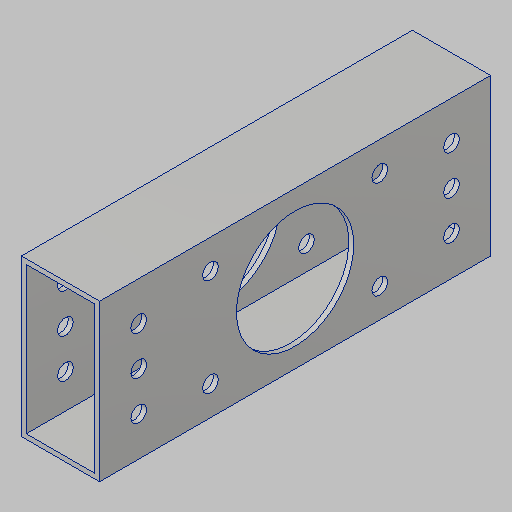
# Autodesk Inventor part: GP5-001
Saved by Autodesk Inventor 2023.4 (Build 274418000, 418)
## iProperties
RuleStatus: InUse
Created: 2025-01-28
Part Number: GP5-001
Material: Aluminum 6061
Document SubType Name: Modeling
Designer: slick
Mass: 304.185 g
Surface Area: 718.547 cm^2
Volume: 112.661 cm^3
Density: 2.7 g/cm^3
Appearance: Aluminum - Flat
AfterDocNew0: SHOW
AfterDocOpen0: SHOW
Author: slick
Autodesk Inventor part; units mm, degrees
ref_plane "YZ Plane" through (0, 0, 0) normal (1, 0, 0) x (0, 1, 0)
ref_plane "XZ Plane" through (0, 0, 0) normal (0, 1, 0) x (-1, 0, 0)
ref_plane "XY Plane" through (0, 0, 0) normal (0, 0, 1) x (1, 0, 0)
sketch "Sketch1" plane through (0, 0, 0) normal (0, 0, 1) x (1, 0, 0)
  line L0 (-12.7, -25.4) -> (12.7, -25.4)
  line L1 (12.7, -25.4) -> (12.7, 25.4)
  line L2 (12.7, 25.4) -> (-12.7, 25.4)
  line L3 (-12.7, 25.4) -> (-12.7, -25.4)
  line L4 (-12.7, -25.4) -> (12.7, 25.4) construction
  line L5 (12.7, -25.4) -> (-12.7, 25.4) construction
  line L6 (-11.1125, 23.8125) -> (11.1125, 23.8125)
  line L7 (11.1125, 23.8125) -> (11.1125, -23.8125)
  line L8 (11.1125, -23.8125) -> (-11.1125, -23.8125)
  line L9 (-11.1125, -23.8125) -> (-11.1125, 23.8125)
  point P0 (0, 0)
  dimension "width" = 25.4
  dimension "height" = 50.8
  dimension "thickness" = 1.5875
  constraints: 20 end point, 4 parallel, 2 midpoint, 2 perpendicular, 1 horizontal, 3 other
  measures "width" distance of L2.end L1.end
  measures "height" distance of L1.end L0.end
  measures "thickness" distance between parallel lines of L2 L6
extrude "Extrusion1" add sketch "Sketch1" along normal mid plane 127
sketch "Sketch2" plane through (-12.7, -25.4, 63.5) normal (-1, 0, 0) x (0, 0, 1)
  circle A0 centre (-63.5, 25.4) radius 31.75 construction
  line L0 (-127, 0) -> (-127, 50.8) projected
  line L1 (-63.5, 50.8) -> (-63.5, 0) construction
  line L2 (0, 0) -> (-127, 0) construction
  line L3 (-127, 50.8) -> (0, 50.8) construction
  point P0 (-63.5, 57.15)
  point P1 (-90.9963, 41.275)
  point P2 (-90.9963, 9.525)
  point P3 (-63.5, -6.35)
  point P4 (-36.0037, 9.525)
  point P5 (-36.0037, 41.275)
  point P6 (-114.3, 38.1)
  point P7 (-114.3, 25.4)
  point P8 (-114.3, 12.7)
  point P9 (-12.7, 38.1)
  point P10 (-12.7, 25.4)
  point P11 (-12.7, 12.7)
  dimension "d5" = 63.5
  dimension "d8" = 360
  dimension "d17" = 12.7
  dimension "d18" = 12.7
  dimension "d19" = 12.7
  constraints: 4 vertical alignment, 3 symmetric about line, 2 end point, 2 midpoint, 1 coincident, 1 horizontal alignment, 9 other
  measures "d17" distance of point (-114.3, 38.1) point (-114.3, 25.4)
  measures "d18" distance of point (-114.3, 12.7) point (-114.3, 25.4)
  measures "d19" distance from line of L0 point (-114.3, 38.1)
hole "Hole1" at (-12.7, 15.875, -27.4963) at (-12.7, -15.875, -27.4963) at (-12.7, -15.875, 27.4963) at (-12.7, 15.875, 27.4963) at (-12.7, 12.7, -50.8) at (-12.7, 0, -50.8) at (-12.7, -12.7, -50.8) at (-12.7, -12.7, 50.8) at (-12.7, 0, 50.8) at (-12.7, 12.7, 50.8) direction (1, 0, 0) diameter 5.1054 end through all clearance for "Flat Head Machine Screw (82)" size "#10" standard "Ansi Unified Screw Threads"
sketch "Sketch3" plane through (12.7, -25.4, 63.5) normal (1, 0, 0) x (0, 0, -1)
  circle A0 centre (63.5, 25.4) radius 19.05
  dimension "d20" = 38.1
  constraints: 1 centre point, 1 coincident
  measures "d20" diameter of A0
extrude "Extrusion2" cut sketch "Sketch3" against normal through all
body "Solid1"
